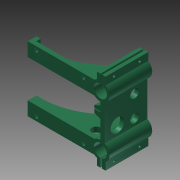
# Autodesk Inventor part: Part10
Saved by Autodesk Inventor 2015 (Build 190159000, 159)
## iProperties
Created: 2015-07-08
Part Number: Part10
Material: ABS Plastic
Document SubType Name: Modeling
Designer: eefred
Density: 1.06 g/cm^3
Appearance: Smooth - Dark Sea Green
Author: eefred
Autodesk Inventor part; units mm, degrees
ref_plane "YZ Plane" through (0, 0, 0) normal (1, 0, 0) x (0, 1, 0)
sketch "Sketch1" plane through (0, 0, 0) normal (0, 1, 0) x (-1, 0, 0)
  line L0 (0, 19.4) -> (0, -19.4)
  line L1 (-5, 20.6533) -> (-5, -20.6533)
  arc A0 (-6, 38.7384) -> (-5, 20.6533) centre (0, 30) ccw
  arc A1 (-2, 37.3321) -> (0, 37.6) centre (0, 30) ccw
  arc A2 (0, 19.4) -> (6.9541, 22) centre (0, 30) ccw
  arc A3 (0, -37.6) -> (-2, -37.3321) centre (0, -30) ccw
  arc A4 (6.9541, -22) -> (0, -19.4) centre (0, -30) ccw
  arc A5 (-5, -20.6533) -> (-6, -38.7384) centre (0, -30) ccw
  line L2 (0, -37.6) -> (0, -47.6)
  line L3 (0, -47.6) -> (4, -47.6)
  line L4 (4, -47.6) -> (4, -39.8163)
  line L5 (-2, -37.3321) -> (-2, -47.6)
  line L6 (-2, -47.6) -> (-6, -47.6)
  line L7 (-6, -47.6) -> (-6, -38.7384)
  line L8 (0, 37.6) -> (0, 47.6)
  line L9 (0, 47.6) -> (4, 47.6)
  line L10 (4, 47.6) -> (4, 39.8163)
  line L11 (-2, 37.3321) -> (-2, 47.6)
  line L12 (-2, 47.6) -> (-6, 47.6)
  line L13 (-6, 47.6) -> (-6, 38.7384)
  arc A6 (6.9541, 38) -> (4, 39.8163) centre (0, 30) ccw
  arc A7 (4, -39.8163) -> (6.9541, -38) centre (0, -30) ccw
  line L14 (6.9541, 38) -> (85, 38)
  line L15 (85, 38) -> (85, 22)
  line L16 (85, 22) -> (6.9541, 22)
  line L17 (6.9541, -22) -> (85, -22)
  line L18 (6.9541, -38) -> (85, -38)
  line L19 (85, -38) -> (85, -22)
  point P0 (0, 0)
  point P1 (0, 0)
  point P2 (85, 30)
  point P3 (85, -30)
  dimension "d5" = 5
  dimension "d6" = 30
  dimension "d7" = 10.6
  dimension "d8" = 7.6
  dimension "d9" = 30
  dimension "d10" = 4
  dimension "d11" = 4
  dimension "d12" = 47.6
  dimension "d13" = 47.6
  dimension "d14" = 2
  dimension "d15" = 2
  dimension "d16" = 4
  dimension "d17" = 4
  dimension "d18" = 16
  dimension "d19" = 16
  dimension "d20" = 85
  dimension "d21" = 85
  constraints: 40 end point, 16 point on circle, 10 perpendicular, 8 centre point, 7 coincident, 6 equal radius, 6 vertical, 4 horizontal, 4 horizontal alignment, 4 vertical alignment, 3 midpoint
  measures "d5" distance between parallel lines of L1 L0
  measures "d6" distance of point (0, 0) A0.centre
  measures "d7" radius of A0
  measures "d8" radius of A1
  measures "d9" distance of point (0, 0) A3.centre
  measures "d10" distance of L2.end L3.end
  measures "d11" distance of L8.end L9.end
  measures "d12" distance from line of point (0, 0) L12
  measures "d13" distance from line of point (0, 0) L6
  measures "d14" distance of L5.end L2.end
  measures "d15" distance of L11.end L8.end
  measures "d16" distance of L5.end L6.end
  measures "d17" distance of L11.end L12.end
  measures "d18" distance of L14.end L15.end
  measures "d19" distance of L18.end L17.end
  measures "d20" distance from line of point (0, 0) L15
  measures "d21" distance from line of point (0, 0) L19
extrude "Extrusion1" add sketch "Sketch1" along normal blind 50
sketch "Sketch2" plane through (2, 0, 47.6) normal (0, 0, 1) x (1, 0, 0)
  circle A0 centre (-82, 90) radius 80
  line L0 (-87, 50) -> (-8.9541, 50) projected
  point P0 (-2, 0)
  dimension "d24" = 160
  dimension "d25" = 80
  dimension "d26" = 40
  constraints: 1 centre point
  measures "d24" diameter of A0
  measures "d25" horizontal distance of point (-2, 0) A0.centre
  measures "d26" distance from line of L0 A0.centre
extrude "Extrusion2" cut sketch "Sketch2" against normal through all
sketch "Sketch3" plane through (-85, 0, 38) normal (0, 0, 1) x (1, 0, 0)
  circle A0 centre (70, 10) radius 5
  line L0 (78.0459, 0) -> (0, 0) projected
  line L1 (85, 0) -> (85, 50) projected
  dimension "d29" = 10
  dimension "d30" = 10
  dimension "d31" = 15
  constraints: 1 centre point
  measures "d29" diameter of A0
  measures "d30" distance from line of L0 A0.centre
  measures "d31" distance from line of L1 A0.centre
extrude "Extrusion3" cut sketch "Sketch3" against normal through all
sketch "Sketch4" plane through (-85, 0, 38) normal (0, 0, 1) x (1, 0, 0)
  line L0 (74.282, 50) -> (78.0459, 50) projected
  line L1 (75, 50) -> (5, 50)
  line L2 (5, 50) -> (5, 5)
  line L3 (5, 5) -> (75, 5)
  line L4 (75, 5) -> (75, 50)
  line L5 (0, 0) -> (0, 10.1564) projected
  line L6 (78.0459, 0) -> (0, 0) projected
  point P0 (85, 0)
  dimension "d34" = 5
  dimension "d35" = 5
  dimension "d36" = 70
  constraints: 8 end point, 2 parallel, 1 horizontal, 1 perpendicular, 1 point on line
  measures "d34" distance between parallel lines of L5 L2
  measures "d35" distance between parallel lines of L6 L3
  measures "d36" distance of L1.start L1.end
extrude "Extrusion4" cut sketch "Sketch4" against normal blind 10
mirror "Mirror1" about plane through (0, 0, 0) normal (0, 0, 1) of "Extrusion4"
sketch "Sketch5" plane through (0, 0, 0) normal (0, -1, 0) x (1, 0, 0)
  circle A0 centre (-75, -33.5) radius 2
  circle A1 centre (-20, -33.5) radius 2
  circle A2 centre (-75, 33.5) radius 2
  circle A3 centre (-20, 33.5) radius 2
  line L0 (0, 19.4) -> (0, -19.4) projected
  point P0 (0, 0)
  dimension "d39" = 4
  dimension "d40" = 20
  dimension "d41" = 55
  dimension "d42" = 33.5
  dimension "d43" = 33.5
  constraints: 4 centre point, 3 equal radius, 2 horizontal alignment, 2 vertical alignment
  measures "d39" diameter of A0
  measures "d40" distance from line of L0 A1.centre
  measures "d41" distance of A0.centre A1.centre
  measures "d42" vertical distance of point (0, 0) A1.centre
  measures "d43" vertical distance of point (0, 0) A3.centre
extrude "Extrusion5" cut sketch "Sketch5" against normal up to next
sketch "Sketch6" plane through (6, 0, 47.6) normal (1, 0, 0) x (0, 0, -1)
  circle A0 centre (4.5, 40) radius 1.4
  circle A1 centre (4.5, 10) radius 1.4
  circle A2 centre (90.7, 40) radius 1.4
  circle A3 centre (90.7, 10) radius 1.4
  circle A4 centre (35.1, 35) radius 5
  circle A5 centre (60.1, 35) radius 5
  circle A6 centre (57.1, 15) radius 8
  line L0 (95.2, 0) -> (95.2, 50) projected
  point P0 (47.6, 0)
  dimension "d46" = 2.8
  dimension "d47" = 86.2
  dimension "d48" = 43.1
  dimension "d49" = 10
  dimension "d50" = 30
  dimension "d51" = 10
  dimension "d52" = 16
  dimension "d53" = 25
  dimension "d54" = 12.5
  dimension "d55" = 35
  dimension "d56" = 15
  dimension "d58" = 9.5
  constraints: 7 centre point, 4 equal radius, 3 horizontal alignment, 2 vertical alignment
  measures "d46" diameter of A0
  measures "d47" distance of A2.centre A0.centre
  measures "d48" horizontal distance of point (47.6, 0) A1.centre
  measures "d49" vertical distance of point (47.6, 0) A1.centre
  measures "d50" distance of A1.centre A0.centre
  measures "d51" diameter of A4
  measures "d52" diameter of A6
  measures "d53" distance of A5.centre A4.centre
  measures "d54" horizontal distance of point (47.6, 0) A4.centre
  measures "d55" vertical distance of point (47.6, 0) A4.centre
  measures "d56" vertical distance of point (47.6, 0) A6.centre
  measures "d58" horizontal distance of point (47.6, 0) A6.centre
extrude "Extrusion6" cut sketch "Sketch6" against normal through all
sketch "Sketch7" plane through (0, 0, 0) normal (0, -1, 0) x (1, 0, 0)
  line L0 (0, 9.5) -> (-7, 9.5)
  line L1 (-7, 9.5) -> (-7, 12.5)
  line L2 (-7, 12.5) -> (0, 15.3)
  line L3 (0, 19.4) -> (0, -19.4) projected
  line L4 (0, 15.3) -> (0, 9.5)
  line L5 (0, 7.6) -> (-7, 7.6)
  line L6 (-7, 7.6) -> (-7, 4.5)
  line L7 (-7, 4.5) -> (0, 1.7)
  line L8 (0, 7.6) -> (0, 1.7)
  line L9 (0, 47.6) -> (-4, 47.6) projected
  point P0 (0, 0)
  dimension "d61" = 7
  dimension "d62" = 1.9
  dimension "d63" = 3.1
  dimension "d64" = 3
  dimension "d65" = 5.8
  dimension "d66" = 5.9
  dimension "d68" = 9.5
  constraints: 16 end point, 5 point on line, 2 collinear, 2 perpendicular, 1 horizontal
  measures "d61" distance of L0.start L0.end
  measures "d62" distance between parallel lines of L5 L0
  measures "d63" distance of L5.end L6.end
  measures "d64" distance of L0.end L1.end
  measures "d65" distance of L2.end L0.start
  measures "d66" distance of L5.start L7.end
  measures "d68" distance from line of point (0, 0) L0
extrude "Extrusion7" add sketch "Sketch7" against normal blind 10
ref_plane "Work Plane1" through (0, 12, 0) normal (0, -1, 0) x (1, 0, 0)
sketch "Sketch8" plane through (0, 12, 0) normal (0, -1, 0) x (1, 0, 0)
  line L0 (0, 9.5) -> (-7, 9.5)
  line L1 (-7, 9.5) -> (-7, 12.5)
  line L2 (-7, 12.5) -> (0, 15.3)
  line L3 (0, 15.3) -> (0, 9.5)
  line L4 (0, 7.6) -> (-7, 7.6)
  line L5 (-7, 7.6) -> (-7, 4.5)
  line L6 (-7, 4.5) -> (0, 1.7)
  line L7 (0, 7.6) -> (0, 1.7)
  point P0 (0, 0)
  dimension "d72" = 7
  dimension "d73" = 1.9
  dimension "d74" = 3.1
  dimension "d75" = 3
  dimension "d76" = 5.8
  dimension "d77" = 5.9
  dimension "d78" = 9.5
  constraints: 16 end point, 2 perpendicular, 2 point on line, 2 vertical alignment, 1 horizontal, 1 vertical
  measures "d72" distance of L0.start L0.end
  measures "d73" distance between parallel lines of L4 L0
  measures "d74" distance of L4.end L5.end
  measures "d75" distance of L0.end L1.end
  measures "d76" distance of L2.end L0.start
  measures "d77" distance of L4.start L6.end
  measures "d78" distance from line of point (0, 0) L0
extrude "Extrusion8" add sketch "Sketch8" against normal blind 11
sketch "Sketch9" plane through (-7, 0, 4.5) normal (-1, 0, 0) x (0, 0, 1)
  line L0 (3.1, 0) -> (4, 0)
  line L1 (4, 0) -> (4, 1)
  line L2 (4, 1) -> (3.1, 1)
  line L3 (3.1, 1) -> (3.1, 0)
  point P0 (-4.5, 0)
  dimension "d81" = 0.9
  dimension "d82" = 1
  constraints: 8 end point, 2 parallel, 1 horizontal, 1 perpendicular
  measures "d81" distance of L2.end L1.end
  measures "d82" distance of L1.end L0.end
extrude "Extrusion9" add sketch "Sketch9" against normal up to next
pattern_linear "Rectangular Pattern1" count 5 spacing 2 along (0, 1, 0) of "Extrusion9"
sketch "Sketch10" plane through (-7, 12, 4.5) normal (-1, 0, 0) x (0, 0, 1)
  line L0 (3.1, 2) -> (4, 2)
  line L1 (4, 2) -> (4, 3)
  line L2 (4, 3) -> (3.1, 3)
  line L3 (3.1, 3) -> (3.1, 2)
  line L4 (0, 0) -> (3.1, 0) projected
  point P0 (-4.5, -12)
  dimension "d91" = 0.9
  dimension "d92" = 1
  dimension "d98" = 2
  constraints: 8 end point, 2 parallel, 1 horizontal, 1 perpendicular, 1 vertical alignment
  measures "d91" distance of L2.end L1.end
  measures "d92" distance of L1.end L0.end
  measures "d98" distance from line of L4 L0.start
extrude "Extrusion10" add sketch "Sketch10" against normal up to next
pattern_linear "Rectangular Pattern3" count 5 spacing 2 along (0, 1, 0) of "Extrusion10"
ref_plane "Work Plane2" through (0, 12, 1.7) normal (0, 0, 1) x (1, 0, 0)
sketch "Sketch11" plane through (0, 12, 1.7) normal (0, 0, 1) x (1, 0, 0)
  line L0 (0, 0) -> (-7, 0)
  line L1 (-7, 0) -> (-7, 2)
  line L2 (-7, 2) -> (0, 0)
  point P0 (0, -12)
  point P1 (0, 0)
  dimension "d102" = 7
  dimension "d103" = 2
  constraints: 6 end point, 4 coincident, 1 horizontal, 1 perpendicular
  measures "d102" distance of L0.start L0.end
  measures "d103" distance of L0.end L1.end
extrude "Extrusion11" cut sketch "Sketch11" along normal blind 14
equation "\"d9\" = d6"
equation "\"d10\" = d11"
equation "\"d13\" = d12"
equation "\"d14\" = d15"
equation "\"d16\" = d11"
equation "\"d17\" = d11"
equation "\"d19\" = d18"
equation "\"d21\" = d20"
equation "\"d43\" = d42"
equation "\"d54\" = 0.5 * d53"
body "Solid1"
